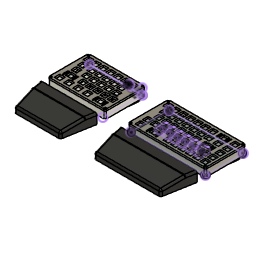
split keyboard v3 (Autodesk Fusion 360 design; units mm, degrees)
Autodesk Fusion 360 part; units mm, degrees
(part 1 of 2)
sketch "스케치1" plane through (0, 0, 0) normal (0, 0, 1) x (1, 0, 0) in component "left-switch"
  line L0 (-176.904915, 103.621) -> (-36.692, 103.621)
  line L1 (-33.692, 100.621) -> (-33.692, 3.272852)
  line L2 (-36.692, 0.272852) -> (-176.904915, 0.272852)
  line L3 (-179.904915, 3.272852) -> (-179.904915, 100.621)
  line L4 (-72.674, 20.2475) -> (-69.474, 20.2475)
  line L5 (-69.474, 20.2475) -> (-69.474, 6.14744)
  line L6 (-69.474, 6.14744) -> (-72.674, 6.14744)
  line L7 (-72.674, 6.14744) -> (-72.674, 20.2475)
  line L8 (-48.874, 20.2475) -> (-45.674, 20.2475)
  line L9 (-45.674, 20.2475) -> (-45.674, 6.14744)
  line L10 (-45.674, 6.14744) -> (-48.874, 6.14744)
  line L11 (-48.874, 6.14744) -> (-48.874, 20.2475)
  line L12 (-170.89943, 20.7987) -> (-156.9992, 20.7987)
  line L13 (-156.9992, 20.7987) -> (-156.9992, 6.89709)
  line L14 (-156.9992, 6.89709) -> (-170.89943, 6.89709)
  line L15 (-170.89943, 6.89709) -> (-170.89943, 20.7987)
  line L16 (-147.0869, 20.7987) -> (-133.1882, 20.7987)
  line L17 (-133.1882, 20.7987) -> (-133.1882, 6.89709)
  line L18 (-133.1882, 6.89709) -> (-147.0869, 6.89709)
  line L19 (-147.0869, 6.89709) -> (-147.0869, 20.7987)
  line L20 (-123.2744, 20.7987) -> (-109.3742, 20.7987)
  line L21 (-109.3742, 20.7987) -> (-109.3742, 6.89709)
  line L22 (-109.3742, 6.89709) -> (-123.2744, 6.89709)
  line L23 (-123.2744, 6.89709) -> (-123.2744, 20.7987)
  line L24 (-99.4619, 20.7987) -> (-85.5631, 20.7987)
  line L25 (-85.5631, 20.7987) -> (-85.5631, 6.89709)
  line L26 (-85.5631, 6.89709) -> (-99.4619, 6.89709)
  line L27 (-99.4619, 6.89709) -> (-99.4619, 20.7987)
  line L28 (-66.124, 20.7987) -> (-52.224, 20.7987)
  line L29 (-52.224, 20.7987) -> (-52.224, 6.89709)
  line L30 (-52.224, 6.89709) -> (-66.124, 6.89709)
  line L31 (-66.124, 6.89709) -> (-66.124, 20.7987)
  line L32 (-167.9242, 39.2977) -> (-164.7244, 39.2977)
  line L33 (-164.7244, 39.2977) -> (-164.7244, 25.1974)
  line L34 (-164.7244, 25.1974) -> (-167.9242, 25.1974)
  line L35 (-167.9242, 25.1974) -> (-167.9242, 39.2977)
  line L36 (-144.1243, 39.2977) -> (-140.9242, 39.2977)
  line L37 (-140.9242, 39.2977) -> (-140.9242, 25.1974)
  line L38 (-140.9242, 25.1974) -> (-144.1243, 25.1974)
  line L39 (-144.1243, 25.1974) -> (-144.1243, 39.2977)
  line L40 (-161.3744, 39.8487) -> (-147.4742, 39.8487)
  line L41 (-147.4742, 39.8487) -> (-147.4742, 25.9471)
  line L42 (-147.4742, 25.9471) -> (-161.3744, 25.9471)
  line L43 (-161.3744, 25.9471) -> (-161.3744, 39.8487)
  line L44 (-130.4181, 39.8487) -> (-116.518, 39.8487)
  line L45 (-116.518, 39.8487) -> (-116.518, 25.9471)
  line L46 (-116.518, 25.9471) -> (-130.4181, 25.9471)
  line L47 (-130.4181, 25.9471) -> (-130.4181, 39.8487)
  line L48 (-111.3681, 39.8487) -> (-97.468, 39.8487)
  line L49 (-97.468, 39.8487) -> (-97.468, 25.9471)
  line L50 (-97.468, 25.9471) -> (-111.3681, 25.9471)
  line L51 (-111.3681, 25.9471) -> (-111.3681, 39.8487)
  line L52 (-92.3181, 39.8487) -> (-78.418, 39.8487)
  line L53 (-78.418, 39.8487) -> (-78.418, 25.9471)
  line L54 (-78.418, 25.9471) -> (-92.3181, 25.9471)
  line L55 (-92.3181, 25.9471) -> (-92.3181, 39.8487)
  line L56 (-73.268, 39.8487) -> (-59.368, 39.8487)
  line L57 (-59.368, 39.8487) -> (-59.368, 25.9471)
  line L58 (-59.368, 25.9471) -> (-73.268, 25.9471)
  line L59 (-73.268, 25.9471) -> (-73.268, 39.8487)
  line L60 (-54.218, 39.8487) -> (-40.318, 39.8487)
  line L61 (-40.318, 39.8487) -> (-40.318, 25.9471)
  line L62 (-40.318, 25.9471) -> (-54.218, 25.9471)
  line L63 (-54.218, 25.9471) -> (-54.218, 39.8487)
  line L64 (-166.1369, 58.8987) -> (-152.238, 58.8987)
  line L65 (-152.238, 58.8987) -> (-152.238, 44.9972)
  line L66 (-152.238, 44.9972) -> (-166.1369, 44.9972)
  line L67 (-166.1369, 44.9972) -> (-166.1369, 58.8987)
  line L68 (-139.9431, 58.8987) -> (-126.043, 58.8987)
  line L69 (-126.043, 58.8987) -> (-126.043, 44.9972)
  line L70 (-126.043, 44.9972) -> (-139.9431, 44.9972)
  line L71 (-139.9431, 44.9972) -> (-139.9431, 58.8987)
  line L72 (-120.8931, 58.8987) -> (-106.993, 58.8987)
  line L73 (-106.993, 58.8987) -> (-106.993, 44.9972)
  line L74 (-106.993, 44.9972) -> (-120.8931, 44.9972)
  line L75 (-120.8931, 44.9972) -> (-120.8931, 58.8987)
  line L76 (-101.8431, 58.8987) -> (-87.943, 58.8987)
  line L77 (-87.943, 58.8987) -> (-87.943, 44.9972)
  line L78 (-87.943, 44.9972) -> (-101.8431, 44.9972)
  line L79 (-101.8431, 44.9972) -> (-101.8431, 58.8987)
  line L80 (-82.7931, 58.8987) -> (-68.893, 58.8987)
  line L81 (-68.893, 58.8987) -> (-68.893, 44.9972)
  line L82 (-68.893, 44.9972) -> (-82.7931, 44.9972)
  line L83 (-82.7931, 44.9972) -> (-82.7931, 58.8987)
  line L84 (-63.743, 58.8987) -> (-49.843, 58.8987)
  line L85 (-49.843, 58.8987) -> (-49.843, 44.9972)
  line L86 (-49.843, 44.9972) -> (-63.743, 44.9972)
  line L87 (-63.743, 44.9972) -> (-63.743, 58.8987)
  line L88 (-168.5182, 77.9473) -> (-154.6179, 77.9473)
  line L89 (-154.6179, 77.9473) -> (-154.6179, 64.0472)
  line L90 (-154.6179, 64.0472) -> (-168.5182, 64.0472)
  line L91 (-168.5182, 64.0472) -> (-168.5182, 77.9473)
  line L92 (-144.7056, 77.9473) -> (-130.8055, 77.9473)
  line L93 (-130.8055, 77.9473) -> (-130.8055, 64.0472)
  line L94 (-130.8055, 64.0472) -> (-144.7056, 64.0472)
  line L95 (-144.7056, 64.0472) -> (-144.7056, 77.9473)
  line L96 (-125.6556, 77.9473) -> (-111.7555, 77.9473)
  line L97 (-111.7555, 77.9473) -> (-111.7555, 64.0472)
  line L98 (-111.7555, 64.0472) -> (-125.6556, 64.0472)
  line L99 (-125.6556, 64.0472) -> (-125.6556, 77.9473)
  line L100 (-106.6056, 77.9473) -> (-92.7055, 77.9473)
  line L101 (-92.7055, 77.9473) -> (-92.7055, 64.0472)
  line L102 (-92.7055, 64.0472) -> (-106.6056, 64.0472)
  line L103 (-106.6056, 64.0472) -> (-106.6056, 77.9473)
  line L104 (-87.5556, 77.9473) -> (-73.655, 77.9473)
  line L105 (-73.655, 77.9473) -> (-73.655, 64.0472)
  line L106 (-73.655, 64.0472) -> (-87.5556, 64.0472)
  line L107 (-87.5556, 64.0472) -> (-87.5556, 77.9473)
  line L108 (-68.507, 77.9473) -> (-54.607, 77.9473)
  line L109 (-54.607, 77.9473) -> (-54.607, 64.0472)
  line L110 (-54.607, 64.0472) -> (-68.507, 64.0472)
  line L111 (-68.507, 64.0472) -> (-68.507, 77.9473)
  line L112 (-173.28068, 96.9973) -> (-159.3804, 96.9973)
  line L113 (-159.3804, 96.9973) -> (-159.3804, 83.0972)
  line L114 (-159.3804, 83.0972) -> (-173.28068, 83.0972)
  line L115 (-173.28068, 83.0972) -> (-173.28068, 96.9973)
  line L116 (-154.2307, 96.9973) -> (-140.3305, 96.9973)
  line L117 (-140.3305, 96.9973) -> (-140.3305, 83.0972)
  line L118 (-140.3305, 83.0972) -> (-154.2307, 83.0972)
  line L119 (-154.2307, 83.0972) -> (-154.2307, 96.9973)
  line L120 (-135.1821, 96.9973) -> (-121.2805, 96.9973)
  line L121 (-121.2805, 96.9973) -> (-121.2805, 83.0972)
  line L122 (-121.2805, 83.0972) -> (-135.1821, 83.0972)
  line L123 (-135.1821, 83.0972) -> (-135.1821, 96.9973)
  line L124 (-116.1321, 96.9973) -> (-102.2305, 96.9973)
  line L125 (-102.2305, 96.9973) -> (-102.2305, 83.0972)
  line L126 (-102.2305, 83.0972) -> (-116.1321, 83.0972)
  line L127 (-116.1321, 83.0972) -> (-116.1321, 96.9973)
  line L128 (-97.0821, 96.9973) -> (-83.1805, 96.9973)
  line L129 (-83.1805, 96.9973) -> (-83.1805, 83.0972)
  line L130 (-83.1805, 83.0972) -> (-97.0821, 83.0972)
  line L131 (-97.0821, 83.0972) -> (-97.0821, 96.9973)
  line L132 (-78.032, 96.9973) -> (-64.132, 96.9973)
  line L133 (-64.132, 96.9973) -> (-64.132, 83.0972)
  line L134 (-64.132, 83.0972) -> (-78.032, 83.0972)
  line L135 (-78.032, 83.0972) -> (-78.032, 96.9973)
  line L136 (-58.981, 96.9973) -> (-45.08, 96.9973)
  line L137 (-45.08, 96.9973) -> (-45.08, 83.0972)
  line L138 (-45.08, 83.0972) -> (-58.981, 83.0972)
  line L139 (-58.981, 83.0972) -> (-58.981, 96.9973)
  arc A0 (-179.904915, 3.272852) -> (-176.904915, 0.272852) centre (-176.904915, 3.272852) ccw
  arc A1 (-176.904915, 103.621) -> (-179.904915, 100.621) centre (-176.904915, 100.621) ccw
  arc A2 (-33.692, 100.621) -> (-36.692, 103.621) centre (-36.692, 100.621) ccw
  arc A3 (-36.692, 0.272852) -> (-33.692, 3.272852) centre (-36.692, 3.272852) ccw
  circle A4 centre (-176.904915, 100.621) radius 1.775
  circle A5 centre (-176.904915, 3.272852) radius 1.775
  circle A6 centre (-36.692, 3.272852) radius 1.775
  circle A7 centre (-36.692, 100.621) radius 1.775
  point P0 (-179.904915, 103.621)
  point P1 (-33.692, 0.272852)
  point P2 (-179.904915, 0.272852)
  dimension "d1" = 103.348148
  dimension "d2" = 146.212915
  dimension "d3" = 13.90161
  dimension "d4" = 13.90023
  dimension "d5" = 179.904915
  dimension "d14" = 3
  dimension "d15" = 3
  dimension "d16" = 3
  dimension "d17" = 3
  dimension "d18" = 3.55
  dimension "d19" = 3.55
  dimension "d20" = 3.55
  dimension "d21" = 3.55
  constraint vertical L3
  constraint horizontal L2
  constraint tangent L3 A0
  constraint tangent L2 A0
  constraint tangent L0 A1
  constraint tangent L3 A1
  constraint tangent L0 A2
  constraint tangent L1 A2
  constraint tangent L1 A3
  constraint tangent L2 A3
  constraint concentric A1 A4
  constraint concentric A0 A5
  constraint concentric A3 A6
  constraint concentric A2 A7
  measures "d14" radius of A0
  measures "d15" radius of A1
  measures "d16" radius of A2
  measures "d17" radius of A3
  measures "d18" diameter of A4
  measures "d19" diameter of A5
  measures "d20" diameter of A6
  measures "d21" diameter of A7
extrude "돌출1" add sketch "스케치1" along normal blind 4.5 contours L0 L1 L2 L3 A0 A1 A2 A3 picked at (-39.696667, 74.5223) makes body 1 in component "left-switch"
sketch "스케치2" plane through (0, 0, 4.5) normal (0, 0, 1) x (-1, 0, 0) in component "left-switch"
  circle A0 centre (176.904915, -100.621) radius 1.775
  circle A1 centre (176.904915, -3.272852) radius 1.775
  circle A2 centre (36.692, -3.272852) radius 1.775
  circle A3 centre (36.692, -100.621) radius 1.775
  circle A4 centre (176.904915, -100.621) radius 3.1
  circle A5 centre (36.692, -100.621) radius 3.1
  circle A6 centre (36.692, -3.272852) radius 3.1
  circle A7 centre (176.904915, -3.272852) radius 3.1
  dimension "d24" = 6.2
  dimension "d25" = 6.2
  dimension "d26" = 6.2
  dimension "d27" = 6.2
  constraint concentric A0 A4
  constraint concentric A3 A5
  constraint concentric A2 A6
  constraint concentric A1 A7
  measures "d24" diameter of A4
  measures "d25" diameter of A5
  measures "d26" diameter of A6
  measures "d27" diameter of A7
extrude "돌출2" cut sketch "스케치2" against normal blind 1.1 contours A4 | A5 | A6 | A7 picked at (175.134258, -102.594321) picked at (35.235227, -98.405816) picked at (39.332183, -3.515046) picked at (175.069433, -5.186025) bodies 1 in component "left-switch"
sketch "스케치1 (2)" plane through (0, 0, 0) normal (0, 0, 1) x (1, 0, 0) in component "left-body"
  line L0 (-179.904915, 3.272852) -> (-179.904915, 100.621)
  arc A0 (-179.904915, 3.272852) -> (-176.904915, 0.272852) centre (-176.904915, 3.272852) ccw
  line L1 (-36.692, 0.272852) -> (-176.904915, 0.272852)
  circle A1 centre (-176.904915, 3.272852) radius 1.775
  arc A2 (-36.692, 0.272852) -> (-33.692, 3.272852) centre (-36.692, 3.272852) ccw
  circle A3 centre (-36.692, 3.272852) radius 1.775
  line L2 (-33.692, 100.621) -> (-33.692, 3.272852)
  arc A4 (-33.692, 100.621) -> (-36.692, 103.621) centre (-36.692, 100.621) ccw
  circle A5 centre (-36.692, 100.621) radius 1.775
  line L3 (-176.904915, 103.621) -> (-36.692, 103.621)
  arc A6 (-176.904915, 103.621) -> (-179.904915, 100.621) centre (-176.904915, 100.621) ccw
  circle A7 centre (-176.904915, 100.621) radius 1.775
  line L4 (-174.404915, 100.621) -> (-39.192, 100.621)
  arc A8 (-176.904915, 98.121) -> (-174.404915, 100.621) centre (-176.904915, 100.621) ccw
  line L5 (-176.904915, 5.772852) -> (-176.904915, 98.121)
  arc A9 (-174.404915, 3.272852) -> (-176.904915, 5.772852) centre (-176.904915, 3.272852) ccw
  arc A10 (-36.692, 5.772852) -> (-39.192, 3.272852) centre (-36.692, 3.272852) ccw
  line L6 (-39.192, 3.272852) -> (-174.404915, 3.272852)
  arc A11 (-39.192, 100.621) -> (-36.692, 98.121) centre (-36.692, 100.621) ccw
  line L7 (-36.692, 98.121) -> (-36.692, 5.772852)
  dimension "d31" = 5
  dimension "d32" = 5
  dimension "d33" = 5
  dimension "d34" = 5
  constraint concentric A6 A8
  constraint concentric A0 A9
  constraint concentric A3 A10
  constraint concentric A4 A11
  measures "d31" diameter of A8
  measures "d32" diameter of A9
  measures "d33" diameter of A10
  measures "d34" diameter of A11
extrude "돌출1'" add sketch "스케치1 (2)" against normal blind 15.8 separate body contours L0 A0 L1 A2 L2 A4 L3 A6 picked at (-129.333944, 102.621) makes body 2 in component "left-body"
sketch "스케치2 (2)" plane through (0, 0, -15.8) normal (0, 0, -1) x (1, 0, 0) in component "left-body"
  line L0 (-179.904915, -3.272852) -> (-179.904915, -100.621)
  arc A0 (-176.904915, -0.272852) -> (-179.904915, -3.272852) centre (-176.904915, -3.272852) ccw
  circle A1 centre (-176.904915, -3.272852) radius 1.775
  line L1 (-36.692, -0.272852) -> (-176.904915, -0.272852)
  arc A2 (-33.692, -3.272852) -> (-36.692, -0.272852) centre (-36.692, -3.272852) ccw
  circle A3 centre (-36.692, -3.272852) radius 1.775
  line L2 (-33.692, -100.621) -> (-33.692, -3.272852)
  arc A4 (-36.692, -103.621) -> (-33.692, -100.621) centre (-36.692, -100.621) ccw
  line L3 (-176.904915, -103.621) -> (-36.692, -103.621)
  arc A5 (-179.904915, -100.621) -> (-176.904915, -103.621) centre (-176.904915, -100.621) ccw
  circle A6 centre (-176.904915, -100.621) radius 1.775
  circle A7 centre (-36.692, -100.621) radius 1.775
  line L4 (-63.743, -44.9972) -> (-63.743, -58.8987)
  line L5 (-68.893, -58.8987) -> (-68.893, -44.9972)
  line L6 (-82.7931, -44.9972) -> (-82.7931, -58.8987)
  line L7 (-87.943, -58.8987) -> (-87.943, -44.9972)
  line L8 (-101.8431, -44.9972) -> (-101.8431, -58.8987)
  line L9 (-106.993, -58.8987) -> (-106.993, -44.9972)
  line L10 (-120.8931, -44.9972) -> (-120.8931, -58.8987)
  line L11 (-126.043, -58.8987) -> (-126.043, -44.9972)
  line L12 (-139.9431, -44.9972) -> (-139.9431, -58.8987)
  line L13 (-152.238, -58.8987) -> (-152.238, -44.9972)
  line L14 (-166.1369, -44.9972) -> (-166.1369, -58.8987)
  line L15 (-63.743, -51.248727) -> (-68.893, -51.248727)
  line L16 (-82.7931, -51.94795) -> (-87.943, -51.94795)
  line L17 (-101.8431, -51.94795) -> (-106.993, -51.94795)
  line L18 (-120.8931, -51.94795) -> (-126.043, -51.94795)
  line L19 (-139.9431, -51.94795) -> (-152.238, -51.94795)
  line L20 (-144.09055, -53.94795) -> (-148.09055, -53.94795)
  line L21 (-148.09055, -53.94795) -> (-148.09055, -49.94795)
  line L22 (-148.09055, -49.94795) -> (-144.09055, -49.94795)
  line L23 (-144.09055, -49.94795) -> (-144.09055, -53.94795)
  line L24 (-144.09055, -53.94795) -> (-148.09055, -49.94795) construction
  line L25 (-148.09055, -53.94795) -> (-144.09055, -49.94795) construction
  line L26 (-121.96805, -53.44795) -> (-124.96805, -53.44795)
  line L27 (-124.96805, -53.44795) -> (-124.96805, -50.44795)
  line L28 (-124.96805, -50.44795) -> (-121.96805, -50.44795)
  line L29 (-121.96805, -50.44795) -> (-121.96805, -53.44795)
  line L30 (-121.96805, -53.44795) -> (-124.96805, -50.44795) construction
  line L31 (-124.96805, -53.44795) -> (-121.96805, -50.44795) construction
  line L32 (-102.91805, -53.44795) -> (-105.91805, -53.44795)
  line L33 (-105.91805, -53.44795) -> (-105.91805, -50.44795)
  line L34 (-105.91805, -50.44795) -> (-102.91805, -50.44795)
  line L35 (-102.91805, -50.44795) -> (-102.91805, -53.44795)
  line L36 (-102.91805, -53.44795) -> (-105.91805, -50.44795) construction
  line L37 (-105.91805, -53.44795) -> (-102.91805, -50.44795) construction
  line L38 (-83.86805, -53.44795) -> (-86.86805, -53.44795)
  line L39 (-86.86805, -53.44795) -> (-86.86805, -50.44795)
  line L40 (-86.86805, -50.44795) -> (-83.86805, -50.44795)
  line L41 (-83.86805, -50.44795) -> (-83.86805, -53.44795)
  line L42 (-83.86805, -53.44795) -> (-86.86805, -50.44795) construction
  line L43 (-86.86805, -53.44795) -> (-83.86805, -50.44795) construction
  line L44 (-64.818, -52.748727) -> (-67.818, -52.748727)
  line L45 (-67.818, -52.748727) -> (-67.818, -49.748727)
  line L46 (-67.818, -49.748727) -> (-64.818, -49.748727)
  line L47 (-64.818, -49.748727) -> (-64.818, -52.748727)
  line L48 (-64.818, -52.748727) -> (-67.818, -49.748727) construction
  line L49 (-67.818, -52.748727) -> (-64.818, -49.748727) construction
  point P0 (-146.09055, -51.94795)
  point P1 (-123.46805, -51.94795)
  point P2 (-104.41805, -51.94795)
  point P3 (-85.36805, -51.94795)
  point P4 (-66.318, -51.248727)
  dimension "d129" = 4
  dimension "d130" = 4
  dimension "d131" = 3
  dimension "d132" = 3
  dimension "d133" = 3
  dimension "d134" = 3
  dimension "d135" = 3
  dimension "d136" = 3
  dimension "d137" = 3
  dimension "d138" = 3
  constraint perpendicular L5 L15
  constraint horizontal L20
  constraint perpendicular L20 L21
  constraint parallel L20 L22
  constraint parallel L21 L23
  constraint horizontal L26
  constraint perpendicular L26 L27
  constraint parallel L26 L28
  constraint parallel L27 L29
  constraint horizontal L32
  constraint perpendicular L32 L33
  constraint parallel L32 L34
  constraint parallel L33 L35
  constraint horizontal L38
  constraint perpendicular L38 L39
  constraint parallel L38 L40
  constraint parallel L39 L41
  constraint horizontal L44
  constraint perpendicular L44 L45
  constraint parallel L44 L46
  constraint parallel L45 L47
extrude "돌출2'" add sketch "스케치2 (2)" along normal blind 2 contours L0 A0 L1 A2 L2 A4 L3 A5 | L15 L44 L45 L47 | L15 L45 L46 L47 | L16 L38 L39 L41 | L16 L39 L40 L41 | L17 L32 L33 L35 | L17 L33 L34 L35 | L18 L26 L27 L29 | L18 L27 L28 L29 | L19 L20 L21 L23 | L19 L21 L22 L23 picked at (-106.504988, -18.545043) picked at (-66.818, -51.748727) picked at (-66.818, -50.248727) picked at (-85.86805, -52.44795) picked at (-85.86805, -50.94795) picked at (-103.91805, -52.94795) picked at (-103.91805, -51.44795) picked at (-122.96805, -52.94795) picked at (-122.96805, -51.44795) picked at (-146.757217, -52.614617) picked at (-145.423883, -50.614617) bodies 2 in component "left-body"
sketch "스케치3" plane through (0, 0, -17.8) normal (0, 0, -1) x (1, 0, 0) in component "left-body"
  circle A0 centre (-36.692, -3.272852) radius 1.775
  circle A1 centre (-176.904915, -3.272852) radius 1.775
  circle A2 centre (-176.904915, -100.621) radius 1.775
  circle A3 centre (-36.692, -100.621) radius 1.775
  circle A4 centre (-176.904915, -3.272852) radius 3.1
  circle A5 centre (-36.692, -3.272852) radius 3.1
  circle A6 centre (-36.692, -100.621) radius 3.1
  circle A7 centre (-176.904915, -100.621) radius 3.1
  dimension "d39" = 6.2
  dimension "d40" = 6.2
  dimension "d41" = 6.2
  dimension "d42" = 6.2
  constraint concentric A1 A4
  constraint concentric A0 A5
  constraint concentric A3 A6
  constraint concentric A2 A7
  measures "d39" diameter of A4
  measures "d40" diameter of A5
  measures "d41" diameter of A6
  measures "d42" diameter of A7
extrude "돌출3" cut sketch "스케치3" against normal blind 1.1 contours A4 | A5 | A6 | A7 picked at (-176.8607, -5.923752) picked at (-34.051817, -3.515046) picked at (-38.736989, -102.308378) picked at (-178.675573, -102.594321) bodies 2 in component "left-body"
ref_plane "작업 평면1" through (-39.692, 51.946926, -7.9) normal (-1, 0, 0) x (0, 1, 0) in component "left-body"
sketch "스케치4" plane through (-39.692, 0, 0) normal (-1, 0, 0) x (0, -1, 0) in component "left-body"
  line L0 (-99.839975, -17.8) -> (-4.053877, -17.8)
  line L1 (-0.272852, -17.8) -> (-99.839975, -17.8)
  line L2 (-99.839975, -17.8) -> (-96.419774, -27.196926)
  line L3 (-0.272852, -17.8) -> (-96.419774, -27.196926)
  point P0 (-0.272852, -17.8)
  point P1 (-103.621, -17.8)
  dimension "d46" = 70
  dimension "d47" = 10
  measures "d46" angle of L1 L2
extrude "돌출4" add sketch "스케치4" along normal blind 134 contours L0 L1 L2 L3 picked at (-66.771209, -20.932309) bodies 2 in component "left-body"
fillet "필렛1" radius 3 1 edges at (-173.692, 98.129874, -22.498463) on bodies 2 in component "left-body"
fillet "필렛2" radius 3 1 edges at (-39.692, 98.129874, -22.498463) on bodies 2 in component "left-body"
sketch "스케치1 (3)" plane through (0, 0, -15.8) normal (0, 0, 1) x (-1, 0, 0)
  line L0 (39.192, -100.621) -> (174.404915, -100.621)
  line L1 (54.192, -87.321) -> (42.192, -87.321)
  line L2 (42.192, -87.321) -> (42.192, -84.321)
  line L3 (42.192, -84.321) -> (54.192, -84.321)
  line L4 (54.192, -84.321) -> (54.192, -87.321)
  line L5 (85.692, -65.221) -> (67.692, -65.221)
  line L6 (67.692, -65.221) -> (67.692, -62.221)
  line L7 (67.692, -62.221) -> (85.692, -62.221)
  line L8 (85.692, -62.221) -> (85.692, -65.221)
  line L9 (39.692, -0.272852) -> (39.692, -99.839975)
  dimension "d54" = 12
  dimension "d55" = 3
  dimension "d56" = 13.3
  dimension "d57" = 3
  dimension "d58" = 18
  dimension "d59" = 3
  dimension "d60" = 35.4
  dimension "d61" = 28
  constraint horizontal L1
  constraint vertical L2
  constraint horizontal L3
  constraint vertical L4
  constraint horizontal L5
  constraint vertical L6
  constraint horizontal L7
  constraint vertical L8
  measures "d54" distance of L1.start L1.end
  measures "d55" distance of L1.start L3.end
  measures "d56" distance of L0 L1
  measures "d57" horizontal distance of L0.start L1.end
  measures "d58" distance of L5.start L5.end
  measures "d59" distance of L5.start L7.end
  measures "d60" distance of L0 L5
  measures "d61" distance of L6 L9
extrude "돌출5" add sketch "스케치1 (3)" along normal blind 2 contours L1 L2 L3 L4 | L5 L6 L7 L8 picked at (50.192, -86.321) picked at (79.692, -64.221) bodies 2 in component "left-body"
sketch "스케치2 (3)" plane through (0, 100.621, 0) normal (0, -1, 0) x (1, 0, 0)
  line L0 (-39.192, -15.8) -> (-174.404915, -15.8)
  line L1 (-39.192, 0) -> (-39.192, -15.8)
  circle A0 centre (-46.192, -12.4) radius 3.2
  line L2 (-79.092, -14.35) -> (-74.192, -14.35)
  arc A1 (-74.192, -14.35) -> (-74.192, -10.65) centre (-74.192, -12.5) ccw
  line L3 (-74.192, -10.65) -> (-79.092, -10.65)
  arc A2 (-79.092, -10.65) -> (-79.092, -14.35) centre (-79.092, -12.5) ccw
  line L4 (-79.092, -12.5) -> (-74.192, -12.5) construction
  line L5 (-54.192, -15.8) -> (-42.192, -15.8)
  line L6 (-42.192, -15.8) -> (-54.192, -15.8)
  line L7 (-85.692, -15.8) -> (-67.692, -15.8)
  line L8 (-67.692, -15.8) -> (-85.692, -15.8)
  line L9 (-39.192, -15.8) -> (-36.692, -15.8)
  line L10 (-39.192, -15.8) -> (-174.404915, -15.8)
  line L11 (-176.904915, -15.8) -> (-174.404915, -15.8)
  line L12 (-176.904915, -15.8) -> (-174.404915, -15.8)
  line L13 (-174.404915, -15.8) -> (-39.192, -15.8)
  line L14 (-39.192, -15.8) -> (-36.692, -15.8)
  dimension "d64" = 6.4
  dimension "d65" = 3.4
  dimension "d66" = 7
  dimension "d67" = 3.7
  dimension "d68" = 3.3
  dimension "d69" = 35
  dimension "d168" = 4.9
  constraint tangent L2 A1
  constraint tangent A1 L3
  constraint parallel L2 L3
  constraint tangent L3 A2
  constraint tangent L2 A2
  constraint horizontal L4
  measures "d64" diameter of A0
  measures "d65" distance of L0 A0.centre
  measures "d66" distance of L1 A0.centre
  measures "d67" diameter of A1
  measures "d68" distance of L0 A1.centre
  measures "d69" distance of L1 A1.centre
  measures "d168" distance of A1.end L3.end
extrude "돌출6" cut sketch "스케치2 (3)" against normal blind 6 contours A0 | L2 A1 L3 A2 picked at (-44.603914, -12.9098) picked at (-75.825333, -13.116667) bodies 2 in component "left-body"
sketch "스케치3 (2)" plane through (0, 103.621, 0) normal (0, 1, 0) x (-1, 0, 0)
  line L0 (74.192, -10.65) -> (79.092, -10.65)
  arc A0 (79.092, -14.35) -> (79.092, -10.65) centre (79.092, -12.5) ccw
  line L1 (79.092, -14.35) -> (74.192, -14.35)
  line L2 (79.092, -8.75) -> (74.192, -8.75)
  arc A1 (74.192, -8.75) -> (74.192, -16.25) centre (74.192, -12.5) ccw
  line L3 (74.192, -16.25) -> (79.092, -16.25)
  arc A2 (79.092, -16.25) -> (79.092, -8.75) centre (79.092, -12.5) ccw
  line L4 (79.092, -12.5) -> (74.192, -12.5) construction
  arc A3 (74.192, -10.65) -> (74.192, -14.35) centre (74.192, -12.5) ccw
  dimension "d72" = 7.5
  constraint tangent L2 A1
  constraint tangent A1 L3
  constraint parallel L2 L3
  constraint tangent L3 A2
  constraint tangent L2 A2
  constraint coincident A1.centre L4.end
  constraint parallel L0 L4
  constraint coincident A0.centre A2.centre
  measures "d72" diameter of A1
extrude "돌출7" cut sketch "스케치3 (2)" against normal blind 1.5 contours L2 A1 L3 A2 picked at (77.458667, -15.616667) bodies 2 in component "left-body"
sketch "스케치1 (4)" plane through (-82.381992, 0, 0) normal (1, 0, 0) x (0, 1, 0) in component "left-palm-rest"
  line L0 (-90, -15) -> (-90, -3)
  line L1 (-90, -3) -> (-44.629745, 5)
  line L2 (-44.629745, 5) -> (-10.090628, 5)
  line L3 (-10.090628, 5) -> (-10, -15)
  line L4 (-10, -15) -> (-90, -15)
extrude "돌출1''" add sketch "스케치1 (4)" along normal blind 146.1125 separate body contours L0 L1 L2 L3 L4 picked at (-48.209915, -8.333333) makes body 3 in component "left-palm-rest"
draft "기울기1" angle -10 neutral plane through (-82.381992, -10.090628, 5) pull (0, 0.99999, 0.004531) 1 faces at (63.730508, -48.209915, -8.333333) on bodies 3 in component "left-palm-rest"
move_body "이동1" bodies 3 to x (1, 0, 0) y (0, 1, 0) z (0, 0, 1) at (-65, 0, 0) in component "left-palm-rest"
draft "기울기2" angle -10 neutral plane through (-147.381992, -10.090628, 5) pull (0, 0.99999, 0.004531) 1 faces at (-147.381992, -48.209915, -8.333333) on bodies 3 in component "left-palm-rest"
fillet "모깎기1" radius 5 8 edges at (-74.325742, -90, -3) (-11.362762, -67.314873, 1) (-74.325742, -44.629745, 5) (-4.31455, -27.360187, 5) (-15.370711, -90, -9) (-144.336934, -27.360187, 5) (-137.288721, -67.314873, 1) (-133.280772, -90, -9) on bodies 3 in component "left-palm-rest"
sketch "스케치1 (5)" plane through (0, 0, 0) normal (0, 0, 1) x (1, 0, 0) in component "right-switch"
  line L0 (3.095085, 103.621) -> (195.695, 103.621)
  line L1 (198.695, 100.621) -> (198.695, 3.272852)
  line L2 (195.695, 0.272852) -> (3.095085, 0.272852)
  line L3 (0.095085, 3.272852) -> (0.095085, 100.621)
  line L4 (40.6506, 20.2475) -> (43.8506, 20.2475)
  line L5 (43.8506, 20.2475) -> (43.8506, 6.14744)
  line L6 (43.8506, 6.14744) -> (40.6506, 6.14744)
  line L7 (40.6506, 6.14744) -> (40.6506, 20.2475)
  line L8 (64.4507, 20.2475) -> (67.6508, 20.2475)
  line L9 (67.6508, 20.2475) -> (67.6508, 6.14744)
  line L10 (67.6508, 6.14744) -> (64.4507, 6.14744)
  line L11 (64.4507, 6.14744) -> (64.4507, 20.2475)
  line L12 (11.4818, 20.7987) -> (25.3821, 20.7987)
  line L13 (25.3821, 20.7987) -> (25.3821, 6.89709)
  line L14 (25.3821, 6.89709) -> (11.4818, 6.89709)
  line L15 (11.4818, 6.89709) -> (11.4818, 20.7987)
  line L16 (47.2006, 20.7987) -> (61.1008, 20.7987)
  line L17 (61.1008, 20.7987) -> (61.1008, 6.89709)
  line L18 (61.1008, 6.89709) -> (47.2006, 6.89709)
  line L19 (47.2006, 6.89709) -> (47.2006, 20.7987)
  line L20 (82.9194, 20.7987) -> (96.8195, 20.7987)
  line L21 (96.8195, 20.7987) -> (96.8195, 6.89709)
  line L22 (96.8195, 6.89709) -> (82.9194, 6.89709)
  line L23 (82.9194, 6.89709) -> (82.9194, 20.7987)
  line L24 (101.969, 20.7987) -> (115.87, 20.7987)
  line L25 (115.87, 20.7987) -> (115.87, 6.89709)
  line L26 (115.87, 6.89709) -> (101.969, 6.89709)
  line L27 (101.969, 6.89709) -> (101.969, 20.7987)
  line L28 (121.019, 20.7987) -> (134.92, 20.7987)
  line L29 (134.92, 20.7987) -> (134.92, 6.89709)
  line L30 (134.92, 6.89709) -> (121.019, 6.89709)
  line L31 (121.019, 6.89709) -> (121.019, 20.7987)
  line L32 (140.069, 20.7987) -> (153.97, 20.7987)
  line L33 (153.97, 20.7987) -> (153.97, 6.89709)
  line L34 (153.97, 6.89709) -> (140.069, 6.89709)
  line L35 (140.069, 6.89709) -> (140.069, 20.7987)
  line L36 (159.119, 20.7987) -> (173.02, 20.7987)
  line L37 (173.02, 20.7987) -> (173.02, 6.89709)
  line L38 (173.02, 6.89709) -> (159.119, 6.89709)
  line L39 (159.119, 6.89709) -> (159.119, 20.7987)
  line L40 (178.169, 20.7987) -> (192.07, 20.7987)
  line L41 (192.07, 20.7987) -> (192.07, 6.89709)
  line L42 (192.07, 6.89709) -> (178.169, 6.89709)
  line L43 (178.169, 6.89709) -> (178.169, 20.7987)
  line L44 (11.4818, 39.8487) -> (25.3821, 39.8487)
  line L45 (25.3821, 39.8487) -> (25.3821, 25.9471)
  line L46 (25.3821, 25.9471) -> (11.4818, 25.9471)
  line L47 (11.4818, 25.9471) -> (11.4818, 39.8487)
  line L48 (30.5318, 39.8487) -> (44.432, 39.8487)
  line L49 (44.432, 39.8487) -> (44.432, 25.9471)
  line L50 (44.432, 25.9471) -> (30.5318, 25.9471)
  line L51 (30.5318, 25.9471) -> (30.5318, 39.8487)
  line L52 (49.5819, 39.8487) -> (63.482, 39.8487)
  line L53 (63.482, 39.8487) -> (63.482, 25.9471)
  line L54 (63.482, 25.9471) -> (49.5819, 25.9471)
  line L55 (49.5819, 25.9471) -> (49.5819, 39.8487)
  line L56 (68.6319, 39.8487) -> (82.532, 39.8487)
  line L57 (82.532, 39.8487) -> (82.532, 25.9471)
  line L58 (82.532, 25.9471) -> (68.6319, 25.9471)
  line L59 (68.6319, 25.9471) -> (68.6319, 39.8487)
  line L60 (87.6819, 39.8487) -> (101.582, 39.8487)
  line L61 (101.582, 39.8487) -> (101.582, 25.9471)
  line L62 (101.582, 25.9471) -> (87.6819, 25.9471)
  line L63 (87.6819, 25.9471) -> (87.6819, 39.8487)
  line L64 (106.732, 39.8487) -> (120.632, 39.8487)
  line L65 (120.632, 39.8487) -> (120.632, 25.9471)
  line L66 (120.632, 25.9471) -> (106.732, 25.9471)
  line L67 (106.732, 25.9471) -> (106.732, 39.8487)
  line L68 (132.926, 39.8487) -> (146.826, 39.8487)
  line L69 (146.826, 39.8487) -> (146.826, 25.9471)
  line L70 (146.826, 25.9471) -> (132.926, 25.9471)
  line L71 (132.926, 25.9471) -> (132.926, 39.8487)
  line L72 (159.119, 39.8487) -> (173.018, 39.8487)
  line L73 (173.018, 39.8487) -> (173.018, 25.9471)
  line L74 (173.018, 25.9471) -> (159.119, 25.9471)
  line L75 (159.119, 25.9471) -> (159.119, 39.8487)
  line L76 (178.169, 39.8487) -> (192.07, 39.8487)
  line L77 (192.07, 39.8487) -> (192.07, 25.9471)
  line L78 (192.07, 25.9471) -> (178.169, 25.9471)
  line L79 (178.169, 25.9471) -> (178.169, 39.8487)
  line L80 (140.662, 58.3477) -> (143.863, 58.3477)
  line L81 (143.863, 58.3477) -> (143.863, 44.2475)
  line L82 (143.863, 44.2475) -> (140.662, 44.2475)
  line L83 (140.662, 44.2475) -> (140.662, 58.3477)
  line L84 (164.462, 58.3477) -> (167.663, 58.3477)
  line L85 (167.663, 58.3477) -> (167.663, 44.2475)
  line L86 (167.663, 44.2475) -> (164.462, 44.2475)
  line L87 (164.462, 44.2475) -> (164.462, 58.3477)
  line L88 (21.0068, 58.8987) -> (34.9071, 58.8987)
  line L89 (34.9071, 58.8987) -> (34.9071, 44.9972)
  line L90 (34.9071, 44.9972) -> (21.0068, 44.9972)
  line L91 (21.0068, 44.9972) -> (21.0068, 58.8987)
  line L92 (40.0569, 58.8987) -> (53.957, 58.8987)
  line L93 (53.957, 58.8987) -> (53.957, 44.9972)
  line L94 (53.957, 44.9972) -> (40.0569, 44.9972)
  line L95 (40.0569, 44.9972) -> (40.0569, 58.8987)
  line L96 (59.1069, 58.8987) -> (73.007, 58.8987)
  line L97 (73.007, 58.8987) -> (73.007, 44.9972)
  line L98 (73.007, 44.9972) -> (59.1069, 44.9972)
  line L99 (59.1069, 44.9972) -> (59.1069, 58.8987)
  line L100 (78.1569, 58.8987) -> (92.057, 58.8987)
  line L101 (92.057, 58.8987) -> (92.057, 44.9972)
  line L102 (92.057, 44.9972) -> (78.1569, 44.9972)
  line L103 (78.1569, 44.9972) -> (78.1569, 58.8987)
  line L104 (97.2069, 58.8987) -> (111.107, 58.8987)
  line L105 (111.107, 58.8987) -> (111.107, 44.9972)
  line L106 (111.107, 44.9972) -> (97.2069, 44.9972)
  line L107 (97.2069, 44.9972) -> (97.2069, 58.8987)
  line L108 (116.257, 58.8987) -> (130.157, 58.8987)
  line L109 (130.157, 58.8987) -> (130.157, 44.9972)
  line L110 (130.157, 44.9972) -> (116.257, 44.9972)
  line L111 (116.257, 44.9972) -> (116.257, 58.8987)
  line L112 (147.213, 58.8987) -> (161.112, 58.8987)
  line L113 (161.112, 58.8987) -> (161.112, 44.9972)
  line L114 (161.112, 44.9972) -> (147.213, 44.9972)
  line L115 (147.213, 44.9972) -> (147.213, 58.8987)
  line L116 (178.169, 58.8987) -> (192.07, 58.8987)
  line L117 (192.07, 58.8987) -> (192.07, 44.9972)
  line L118 (192.07, 44.9972) -> (178.169, 44.9972)
  line L119 (178.169, 44.9972) -> (178.169, 58.8987)
  line L120 (16.2443, 77.9473) -> (30.1446, 77.9473)
  line L121 (30.1446, 77.9473) -> (30.1446, 64.0472)
  line L122 (30.1446, 64.0472) -> (16.2443, 64.0472)
  line L123 (16.2443, 64.0472) -> (16.2443, 77.9473)
  line L124 (35.2944, 77.9473) -> (49.1945, 77.9473)
  line L125 (49.1945, 77.9473) -> (49.1945, 64.0472)
  line L126 (49.1945, 64.0472) -> (35.2944, 64.0472)
  line L127 (35.2944, 64.0472) -> (35.2944, 77.9473)
  line L128 (54.3444, 77.9473) -> (68.2445, 77.9473)
  line L129 (68.2445, 77.9473) -> (68.2445, 64.0472)
  line L130 (68.2445, 64.0472) -> (54.3444, 64.0472)
  line L131 (54.3444, 64.0472) -> (54.3444, 77.9473)
  line L132 (73.3944, 77.9473) -> (87.2945, 77.9473)
  line L133 (87.2945, 77.9473) -> (87.2945, 64.0472)
  line L134 (87.2945, 64.0472) -> (73.3944, 64.0472)
  line L135 (73.3944, 64.0472) -> (73.3944, 77.9473)
  line L136 (92.4444, 77.9473) -> (106.345, 77.9473)
  line L137 (106.345, 77.9473) -> (106.345, 64.0472)
  line L138 (106.345, 64.0472) -> (92.4444, 64.0472)
  line L139 (92.4444, 64.0472) -> (92.4444, 77.9473)
  line L140 (111.493, 77.9473) -> (125.393, 77.9473)
  line L141 (125.393, 77.9473) -> (125.393, 64.0472)
  line L142 (125.393, 64.0472) -> (111.493, 64.0472)
  line L143 (111.493, 64.0472) -> (111.493, 77.9473)
  line L144 (130.544, 77.9473) -> (144.445, 77.9473)
  line L145 (144.445, 77.9473) -> (144.445, 64.0472)
  line L146 (144.445, 64.0472) -> (130.544, 64.0472)
  line L147 (130.544, 64.0472) -> (130.544, 77.9473)
  line L148 (154.357, 77.9473) -> (168.257, 77.9473)
  line L149 (168.257, 77.9473) -> (168.257, 64.0472)
  line L150 (168.257, 64.0472) -> (154.357, 64.0472)
  line L151 (154.357, 64.0472) -> (154.357, 77.9473)
  line L152 (178.169, 77.9473) -> (192.07, 77.9473)
  line L153 (192.07, 77.9473) -> (192.07, 64.0472)
  line L154 (192.07, 64.0472) -> (178.169, 64.0472)
  line L155 (178.169, 64.0472) -> (178.169, 77.9473)
  line L156 (143.044, 96.4477) -> (146.243, 96.4477)
  line L157 (146.243, 96.4477) -> (146.243, 82.3475)
  line L158 (146.243, 82.3475) -> (143.044, 82.3475)
  line L159 (143.044, 82.3475) -> (143.044, 96.4477)
  line L160 (166.844, 96.4477) -> (170.045, 96.4477)
  line L161 (170.045, 96.4477) -> (170.045, 82.3475)
  line L162 (170.045, 82.3475) -> (166.844, 82.3475)
  line L163 (166.844, 82.3475) -> (166.844, 96.4477)
  line L164 (6.71932, 96.9973) -> (20.6196, 96.9973)
  line L165 (20.6196, 96.9973) -> (20.6196, 83.0972)
  line L166 (20.6196, 83.0972) -> (6.71932, 83.0972)
  line L167 (6.71932, 83.0972) -> (6.71932, 96.9973)
  line L168 (25.7693, 96.9973) -> (39.6695, 96.9973)
  line L169 (39.6695, 96.9973) -> (39.6695, 83.0972)
  line L170 (39.6695, 83.0972) -> (25.7693, 83.0972)
  line L171 (25.7693, 83.0972) -> (25.7693, 96.9973)
  line L172 (44.8179, 96.9973) -> (58.7195, 96.9973)
  line L173 (58.7195, 96.9973) -> (58.7195, 83.0972)
  line L174 (58.7195, 83.0972) -> (44.8179, 83.0972)
  line L175 (44.8179, 83.0972) -> (44.8179, 96.9973)
  line L176 (63.8679, 96.9973) -> (77.7695, 96.9973)
  line L177 (77.7695, 96.9973) -> (77.7695, 83.0972)
  line L178 (77.7695, 83.0972) -> (63.8679, 83.0972)
  line L179 (63.8679, 83.0972) -> (63.8679, 96.9973)
  line L180 (82.9179, 96.9973) -> (96.8195, 96.9973)
  line L181 (96.8195, 96.9973) -> (96.8195, 83.0972)
  line L182 (96.8195, 83.0972) -> (82.9179, 83.0972)
  line L183 (82.9179, 83.0972) -> (82.9179, 96.9973)
  line L184 (101.968, 96.9973) -> (115.868, 96.9973)
  line L185 (115.868, 96.9973) -> (115.868, 83.0972)
  line L186 (115.868, 83.0972) -> (101.968, 83.0972)
  line L187 (101.968, 83.0972) -> (101.968, 96.9973)
  line L188 (121.019, 96.9973) -> (134.92, 96.9973)
  line L189 (134.92, 96.9973) -> (134.92, 83.0972)
  line L190 (134.92, 83.0972) -> (121.019, 83.0972)
  line L191 (121.019, 83.0972) -> (121.019, 96.9973)
  line L192 (149.594, 96.9973) -> (163.493, 96.9973)
  line L193 (163.493, 96.9973) -> (163.493, 83.0972)
  line L194 (163.493, 83.0972) -> (149.594, 83.0972)
  line L195 (149.594, 83.0972) -> (149.594, 96.9973)
  line L196 (178.169, 96.9973) -> (192.068, 96.9973)
  line L197 (192.068, 96.9973) -> (192.068, 83.0972)
  line L198 (192.068, 83.0972) -> (178.169, 83.0972)
  line L199 (178.169, 83.0972) -> (178.169, 96.9973)
  arc A0 (0.095085, 3.272852) -> (3.095085, 0.272852) centre (3.095085, 3.272852) ccw
  arc A1 (3.095085, 103.621) -> (0.095085, 100.621) centre (3.095085, 100.621) ccw
  arc A2 (198.695, 100.621) -> (195.695, 103.621) centre (195.695, 100.621) ccw
  arc A3 (195.695, 0.272852) -> (198.695, 3.272852) centre (195.695, 3.272852) ccw
  circle A4 centre (3.095085, 100.621) radius 1.775
  circle A5 centre (3.095085, 3.272852) radius 1.775
  circle A6 centre (195.695, 3.272852) radius 1.775
  circle A7 centre (195.695, 100.621) radius 1.775
  dimension "d75" = 3
  dimension "d76" = 3
  dimension "d77" = 3
  dimension "d78" = 3
  dimension "d79" = 3.55
  dimension "d80" = 3.55
  dimension "d81" = 3.55
  dimension "d82" = 3.55
  constraint vertical L3
  constraint horizontal L2
  constraint tangent L3 A0
  constraint tangent L2 A0
  constraint tangent L0 A1
  constraint tangent L3 A1
  constraint tangent L0 A2
  constraint tangent L1 A2
  constraint tangent L1 A3
  constraint tangent L2 A3
  constraint concentric A1 A4
  constraint concentric A0 A5
  constraint concentric A3 A6
  constraint concentric A2 A7
  measures "d75" radius of A0
  measures "d76" radius of A1
  measures "d77" radius of A2
  measures "d78" radius of A3
  measures "d79" diameter of A4
  measures "d80" diameter of A5
  measures "d81" diameter of A6
  measures "d82" diameter of A7
extrude "돌출1'''" add sketch "스케치1 (5)" along normal blind 4.5 separate body contours L0 L1 L2 L3 A0 A1 A2 A3 picked at (72.740333, 11.097343) makes body 4 in component "right-switch"
sketch "스케치2 (4)" plane through (0, 0, 4.5) normal (0, 0, 1) x (-1, 0, 0) in component "right-switch"
  circle A0 centre (-3.095085, -100.621) radius 1.775
  circle A1 centre (-3.095085, -3.272852) radius 1.775
  circle A2 centre (-195.695, -3.272852) radius 1.775
  circle A3 centre (-195.695, -100.621) radius 1.775
  circle A4 centre (-3.095085, -100.621) radius 3.1
  circle A5 centre (-3.095085, -3.272852) radius 3.1
  circle A6 centre (-195.695, -3.272852) radius 3.1
  circle A7 centre (-195.695, -100.621) radius 3.1
  dimension "d85" = 6.2
  dimension "d86" = 6.2
  dimension "d87" = 6.2
  dimension "d88" = 6.2
  constraint concentric A0 A4
  constraint concentric A1 A5
  constraint concentric A2 A6
  constraint concentric A3 A7
  measures "d85" diameter of A4
  measures "d86" diameter of A5
  measures "d87" diameter of A6
  measures "d88" diameter of A7
extrude "돌출2''" cut sketch "스케치2 (4)" against normal blind 1.1 contours A4 | A5 | A6 | A7 picked at (-1.638312, -98.405816) picked at (-0.448293, -3.426862) picked at (-195.650785, -5.923752) picked at (-197.795125, -102.23924) bodies 4 in component "right-switch"
sketch "스케치1 (6)" plane through (0, 0, 0) normal (0, 0, -1) x (1, 0, 0) in component "right-body"
  line L0 (28.095085, -103.621) -> (220.695, -103.621)
  arc A0 (220.695, -103.621) -> (223.695, -100.621) centre (220.695, -100.621) ccw
  line L1 (223.695, -100.621) -> (223.695, -3.272852)
  arc A1 (223.695, -3.272852) -> (220.695, -0.272852) centre (220.695, -3.272852) ccw
  circle A2 centre (220.695, -3.272852) radius 1.775
  circle A3 centre (220.695, -100.621) radius 1.775
  circle A4 centre (28.095085, -100.621) radius 1.775
  arc A5 (25.095085, -100.621) -> (28.095085, -103.621) centre (28.095085, -100.621) ccw
  line L2 (25.095085, -3.272852) -> (25.095085, -100.621)
  circle A6 centre (28.095085, -3.272852) radius 1.775
  arc A7 (28.095085, -0.272852) -> (25.095085, -3.272852) centre (28.095085, -3.272852) ccw
  line L3 (220.695, -0.272852) -> (28.095085, -0.272852)
  line L4 (218.195, -3.272852) -> (30.595085, -3.272852)
  arc A8 (220.695, -98.121) -> (218.195, -100.621) centre (220.695, -100.621) ccw
  line L5 (220.695, -100.621) -> (220.695, -98.846)
  line L6 (220.695, -98.121) -> (220.695, -5.772852)
  arc A9 (218.195, -3.272852) -> (220.695, -5.772852) centre (220.695, -3.272852) ccw
  arc A10 (30.595085, -100.621) -> (28.095085, -98.121) centre (28.095085, -100.621) ccw
  line L7 (30.595085, -100.621) -> (218.195, -100.621)
  arc A11 (28.095085, -5.772852) -> (30.595085, -3.272852) centre (28.095085, -3.272852) ccw
  line L8 (28.095085, -5.772852) -> (28.095085, -98.121)
  dimension "d92" = 5
  dimension "d93" = 5
  dimension "d94" = 5
  dimension "d95" = 5
  constraint concentric A3 A8
  constraint coincident A8.start L5
  constraint coincident A3 L5.end
  constraint collinear L5 L6
  constraint concentric A2 A9
  constraint concentric A4 A10
  constraint concentric A7 A11
  measures "d92" diameter of A8
  measures "d93" diameter of A9
  measures "d94" diameter of A10
  measures "d95" diameter of A11
sketch "스케치2 (5)" plane through (0, 0, 0) normal (0, 0, -1) x (1, 0, 0) in component "right-body"
extrude "돌출1''''" add sketch "스케치1 (6)" along normal blind 15.8 separate body contours L0 A0 L1 A1 A5 L2 A7 L3 picked at (93.12839, -102.621) makes body 5 in component "right-body"
sketch "스케치3 (3)" plane through (0, 0, -15.8) normal (0, 0, -1) x (1, 0, 0) in component "right-body"
  line L0 (25.095085, -3.272852) -> (25.095085, -100.621)
  arc A0 (28.095085, -0.272852) -> (25.095085, -3.272852) centre (28.095085, -3.272852) ccw
  line L1 (220.695, -0.272852) -> (28.095085, -0.272852)
  circle A1 centre (28.095085, -3.272852) radius 1.775
  circle A2 centre (220.695, -3.272852) radius 1.775
  arc A3 (223.695, -3.272852) -> (220.695, -0.272852) centre (220.695, -3.272852) ccw
  line L2 (223.695, -100.621) -> (223.695, -3.272852)
  arc A4 (220.695, -103.621) -> (223.695, -100.621) centre (220.695, -100.621) ccw
  circle A5 centre (220.695, -100.621) radius 1.775
  line L3 (28.095085, -103.621) -> (220.695, -103.621)
  arc A6 (25.095085, -100.621) -> (28.095085, -103.621) centre (28.095085, -100.621) ccw
  circle A7 centre (28.095085, -100.621) radius 1.775
  line L4 (117.057, -58.8987) -> (117.057, -44.9972)
  line L5 (122.2069, -44.9972) -> (122.2069, -58.8987)
  line L6 (136.107, -58.8987) -> (136.107, -44.9972)
  line L7 (141.257, -44.9972) -> (141.257, -58.8987)
  line L8 (155.157, -58.8987) -> (155.157, -44.9972)
  line L9 (165.662, -44.2475) -> (165.662, -58.3477)
  line L10 (98.007, -58.8987) -> (98.007, -44.9972)
  line L11 (103.1569, -44.9972) -> (103.1569, -58.8987)
  line L12 (78.957, -58.8987) -> (78.957, -44.9972)
  line L13 (84.1069, -44.9972) -> (84.1069, -58.8987)
  line L14 (65.0569, -44.9972) -> (65.0569, -58.8987)
  line L15 (59.9071, -58.8987) -> (59.9071, -44.9972)
  line L16 (59.9071, -51.94795) -> (65.0569, -51.94795)
  line L17 (78.957, -51.94795) -> (84.1069, -51.94795)
  line L18 (98.007, -51.94795) -> (103.1569, -51.94795)
  line L19 (117.057, -51.94795) -> (122.2069, -51.94795)
  line L20 (136.107, -51.94795) -> (141.257, -51.94795)
  line L21 (155.157, -51.94795) -> (165.662, -51.94795)
  circle A8 centre (62.482, -51.94795) radius 1.5
  circle A9 centre (81.53195, -51.94795) radius 1.5
  circle A10 centre (100.58195, -51.94795) radius 1.5
  circle A11 centre (119.63195, -51.94795) radius 1.5
  circle A12 centre (138.682, -51.94795) radius 1.5
  circle A13 centre (160.4095, -51.94795) radius 2
  point P0 (223.695, -3.272852)
  dimension "d119" = 3
  dimension "d120" = 3
  dimension "d121" = 3
  dimension "d122" = 3
  dimension "d123" = 3
  dimension "d124" = 4
  constraint perpendicular L9 L21
  measures "d119" diameter of A8
  measures "d120" diameter of A9
  measures "d121" diameter of A10
  measures "d122" diameter of A11
  measures "d123" diameter of A12
  measures "d124" diameter of A13
extrude "돌출2'''" add sketch "스케치3 (3)" along normal blind 2 contours L0 A0 L1 A3 L2 A4 L3 A6 | L16 A8 | L16 A8 | L17 A9 | L17 A9 | L18 A10 | L18 A10 | L19 A11 | L19 A11 | L20 A12 | L20 A12 | L21 A13 | L21 A13 picked at (122.83114, -18.250177) picked at (62.848526, -51.313108) picked at (62.83111, -52.837468) picked at (81.0749, -51.374827) picked at (81.464621, -52.726877) picked at (100.1249, -51.374827) picked at (100.514621, -52.726877) picked at (119.1749, -51.374827) picked at (119.564621, -52.726877) picked at (138.864671, -51.333471) picked at (138.499329, -52.562429) picked at (160.076167, -50.619506) picked at (160.014042, -53.354295) bodies 5 in component "right-body"
sketch "스케치5" plane through (0, 0, -17.8) normal (0, 0, -1) x (1, 0, 0) in component "right-body"
  circle A0 centre (220.695, -100.621) radius 1.775
  circle A1 centre (28.095085, -100.621) radius 1.775
  circle A2 centre (28.095085, -3.272852) radius 1.775
  circle A3 centre (220.695, -3.272852) radius 1.775
  circle A4 centre (220.695, -3.272852) radius 3.1
  circle A5 centre (220.607436, -100.621) radius 0.087564
  circle A6 centre (220.695, -100.621) radius 3.1
  circle A7 centre (28.095085, -100.621) radius 3.1
  circle A8 centre (28.095085, -3.272852) radius 3.1
  dimension "d101" = 6.2
  dimension "d102" = 6.2
  dimension "d103" = 6.2
  dimension "d104" = 6.2
  constraint concentric A3 A4
  constraint coincident A0.centre A5
  constraint concentric A0 A6
  constraint concentric A1 A7
  constraint concentric A2 A8
  measures "d101" diameter of A4
  measures "d102" diameter of A6
  measures "d103" diameter of A7
  measures "d104" diameter of A8
extrude "돌출3'" cut sketch "스케치5" against normal blind 1.1 contours A4 | A6 | A7 | A8 picked at (218.859518, -5.186025) picked at (220.739215, -103.2719) picked at (25.454901, -100.378806) picked at (30.741876, -3.426862) bodies 5 in component "right-body"
ref_plane "작업 평면2" through (217.495, 51.946926, -8.9) normal (1, 0, 0) x (0, -1, 0) in component "right-body"
sketch "스케치6" plane through (217.495, 0, 0) normal (1, 0, 0) x (0, 1, 0) in component "right-body"
  line L0 (96.419774, -27.196926) -> (99.839975, -17.8)
  line L1 (99.839975, -17.8) -> (0.272852, -17.8)
  line L2 (0.272852, -17.8) -> (96.419774, -27.196926)
  point P0 (96.419774, -27.196926)
  point P1 (99.839975, -17.8)
  point P2 (0.272852, -17.8)
extrude "돌출4'" add sketch "스케치6" against normal blind 186 contours L0 L1 L2 picked at (65.510867, -20.932309) bodies 5 in component "right-body"
fillet "필렛1'" radius 3 2 edges at (31.495, 98.129874, -22.498463) (217.495, 98.129874, -22.498463) on bodies 5 in component "right-body"
extrude "돌출9" add sketch "스케치2 (2)" against normal blind 15.8 contours L15 L44 L45 L47 | L15 L45 L46 L47 | L16 L38 L39 L41 | L16 L39 L40 L41 | L17 L32 L33 L35 | L17 L33 L34 L35 | L18 L26 L27 L29 | L18 L27 L28 L29 | L19 L20 L21 L23 | L19 L21 L22 L23 picked at (-66.818, -51.748727) picked at (-66.818, -50.248727) picked at (-85.86805, -52.44795) picked at (-85.86805, -50.94795) picked at (-103.91805, -52.94795) picked at (-103.91805, -51.44795) picked at (-122.96805, -52.94795) picked at (-122.96805, -51.44795) picked at (-146.757217, -52.614617) picked at (-145.423883, -50.614617) bodies 2 in component "left-body"